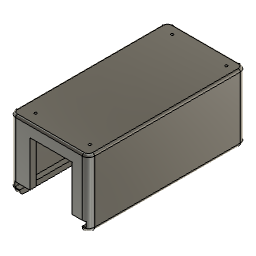
Accelerator UTP v8 (Autodesk Fusion 360 design; units mm, degrees)
Autodesk Fusion 360 part; units mm, degrees
sketch "base" plane through (0, 0, 0) normal (0, 0, 1) x (1, 0, 0) in component "Accelerator"
  line L0 (0, 0) -> (38.5, 0)
  line L1 (38.5, 0) -> (38.5, 74)
  line L2 (38.5, 74) -> (0, 74)
  line L3 (0, 74) -> (0, 0)
  line L4 (0, 59) -> (38.5, 59)
  line L5 (0, 19) -> (38.5, 19)
  line L6 (5, 0) -> (5, 74)
  line L7 (35.5, 0) -> (35.5, 74)
  line L8 (5, 0) -> (7, 5.75) construction
  line L9 (35.5, 0) -> (33.5, 5.75) construction
  point P0 (7, 5.75)
  point P1 (33.5, 5.75)
  point P2 (33.5, 72.25)
  point P3 (7, 72.25)
  dimension "d1" = 26.5
  dimension "d2" = 66.5
  dimension "d4" = 74
  dimension "d9" = 19
  dimension "d33" = 5
  dimension "d34" = 3
  dimension "d101" = 5.75
  dimension "d102" = 40
  dimension "d150" = 38.5
  constraint horizontal L0
  constraint vertical L1
  constraint horizontal L2
  constraint vertical L3
  constraint coincident L0.start L3.end
  constraint horizontal P2 P3
  constraint vertical P0 P3
  constraint horizontal P0 P1
  constraint vertical P1 P2
  constraint coincident L3 L4.start
  constraint coincident L1 L4.end
  constraint perpendicular L1 L4
  constraint coincident L3 L5.start
  constraint coincident L1 L5.end
  constraint perpendicular L1 L5
  constraint coincident L0 L6.start
  constraint coincident L2 L6.end
  constraint coincident L0 L7.start
  constraint coincident L2 L7.end
  constraint perpendicular L2 L7
  constraint vertical L6
  constraint coincident P0 L8.end
  constraint coincident P1 L9.end
  constraint equal L8 L9
  measures "d1" distance of P0 P1
  measures "d2" distance of P0 P3
  measures "d4" distance of L0.end L1.end
  measures "d9" distance of L0.end L5.end
  measures "d33" distance of L0.start L6.start
  measures "d34" distance of L0.end L7.start
  measures "d101" vertical distance of L0.start L8.end
  measures "d102" distance of L4.end L5.end
  measures "d150" distance of L1.end L2.end
extrude "Extrude1" add sketch "base" against normal blind 6 contours L0 L5 L6 L7 | L2 L4 L6 L7 makes body 1 at (25.3333, 6.3333, 0) makes body 2 at (25.3333, 64, 0) in component "Accelerator"
extrude "Extrude2" add sketch "base" against normal blind 3 contours L4 L5 L6 L7 bodies 1 2 in component "Accelerator"
extrude "Extrude3" add sketch "base" against normal blind 33 contours L0 L3 L5 L6 | L3 L4 L5 L6 | L0 L1 L5 L7 | L2 L3 L4 L6 | L1 L4 L5 L7 | L1 L2 L4 L7 bodies 1 in component "Accelerator"
hole "Hole1" at (7, 5.75, 0) at (33.5, 5.75, 0) at (7, 72.25, 0) at (33.5, 72.25, 0) direction (0, 0, -1) diameter 1.2 end up to surface (6 mm away) bodies 1 in component "Accelerator"
sketch "bolts" plane through (5, 0, 0) normal (1, 0, 0) x (0, 1, 0) in component "Accelerator"
  line L0 (19, -6) -> (0, -6)
  line L1 (0, -6) -> (0, -33)
  line L2 (0, -33) -> (74, -33)
  line L3 (74, -33) -> (74, -6)
  line L4 (74, -6) -> (59, -6)
  line L5 (59, -6) -> (59, -3)
  line L6 (59, -3) -> (19, -3)
  line L7 (19, -3) -> (19, -6)
  line L8 (0, -33) -> (17, -11) construction
  line L9 (74, -33) -> (57, -11) construction
  line L10 (74, 0) -> (0, 0)
  point P0 (17, -11)
  point P1 (57, -11)
  dimension "d53" = 11
  dimension "d54" = 40
  constraint coincident L1.end L2.start
  constraint coincident P0 L8.end
  constraint coincident L2.end L3.start
  constraint coincident P1 L9.end
  constraint equal L8 L9
  constraint horizontal P0 P1
  measures "d53" distance of P1 L10
  measures "d54" distance of P0 P1
hole "Hole3" at (5, 17, -11) at (5, 57, -11) direction (-1, 0, 0) diameter 5.3 end up to surface (5 mm away) counterbore diameter 10 counterbore depth 3.5 bodies 1 in component "Accelerator"
fillet "Fillet9" radius 6 2 edges at (20.25, 19, -6) (20.25, 59, -6) on bodies 1 in component "Accelerator"
sketch "flatcable-plate" plane through (0, 74, 0) normal (0, 1, 0) x (-1, 0, 0) in component "Accelerator"
  line L0 (0, 0) -> (-38.5, 0)
  line L1 (-38.5, 0) -> (-38.5, -33)
  line L2 (-38.5, -33) -> (-35.5, -33)
  line L3 (-35.5, -33) -> (-35.5, -6)
  line L4 (-35.5, -6) -> (-5, -6)
  line L5 (-5, -6) -> (-5, -33)
  line L6 (-5, -33) -> (0, -33)
  line L7 (0, -33) -> (0, 0)
  line L8 (-38.5, 0) -> (0, 0)
  line L9 (0, 0) -> (0, -33)
  line L10 (0, -33) -> (-38.5, -33)
  line L11 (-38.5, -33) -> (-38.5, 0)
  constraint horizontal L8
  constraint vertical L9
  constraint horizontal L10
  constraint vertical L11
  constraint coincident L6.end L7.start
  constraint coincident L0.end L1.start
extrude "Extrude12" add sketch "flatcable-plate" along normal blind 3 bodies 1 in component "Accelerator"
sketch "lid-uitsnede" plane through (0, 0, 0) normal (0, -1, 0) x (1, 0, 0) in component "Accelerator"
  line L0 (38.5, 0) -> (0, 0)
  line L1 (0, 0) -> (0, -33)
  line L2 (0, -33) -> (5, -33)
  line L3 (5, -33) -> (5, -6)
  line L4 (5, -6) -> (35.5, -6)
  line L5 (35.5, -6) -> (35.5, -33)
  line L6 (35.5, -33) -> (38.5, -33)
  line L7 (38.5, -33) -> (38.5, 0)
  line L8 (2.5, -28.1) -> (37, -28.1)
  line L9 (37, -28.1) -> (37, -30.5)
  line L10 (37, -30.5) -> (2.5, -30.5)
  line L11 (2.5, -30.5) -> (2.5, -28.1)
  line L12 (2.5, -30.5) -> (0, -33) construction
  line L13 (2.5, -30.5) -> (5, -33) construction
  line L14 (37, -30.5) -> (35.5, -33) construction
  line L15 (37, -30.5) -> (38.5, -33) construction
  dimension "d95" = 2.4
  dimension "d97" = 2.5
  constraint horizontal L8
  constraint vertical L9
  constraint horizontal L10
  constraint vertical L11
  constraint coincident L1.end L2.start
  constraint coincident L2.end L3.start
  constraint coincident L5.end L6.start
  constraint coincident L6.end L7.start
  constraint equal L14 L15
  constraint equal L12 L13
  measures "d95" distance of L8.end L9.end
  measures "d97" vertical distance of L10.end L1.end
sketch "flatcable" plane through (0, 74, 0) normal (0, -1, 0) x (1, 0, 0) in component "Accelerator"
  line L0 (35.5, -33) -> (35.5, -6)
  line L1 (35.5, -6) -> (5, -6)
  line L2 (5, -6) -> (5, -33)
  line L3 (5, -33) -> (35.5, -33)
  line L4 (10.25, -10) -> (30.25, -10)
  line L5 (30.25, -10) -> (30.25, -18.5)
  line L6 (30.25, -18.5) -> (10.25, -18.5)
  line L7 (10.25, -18.5) -> (10.25, -10)
  line L8 (35.5, -33) -> (30.25, -18.5) construction
  line L9 (35.5, -6) -> (30.25, -10) construction
  line L10 (10.25, -10) -> (5, -6) construction
  point P0 (5, -6)
  point P1 (35.5, -6)
  point P2 (35.5, -33)
  dimension "d147" = 20
  dimension "d148" = 8.5
  dimension "d149" = 4
  constraint horizontal L4
  constraint vertical L5
  constraint horizontal L6
  constraint vertical L7
  constraint coincident P2 L0.start
  constraint coincident P1 L0.end
  constraint coincident P0 L1.end
  constraint equal L9 L10
  measures "d147" distance of L4.start L4.end
  measures "d148" distance of L4.start L6.end
  measures "d149" vertical distance of L4.end P1
sketch "space" plane through (0, 0, -6) normal (0, 0, -1) x (1, 0, 0) in component "Accelerator"
  line L0 (5, -13.8038) -> (35.5, -13.8038)
  line L1 (35.5, -13.8038) -> (35.5, 0)
  line L2 (35.5, 0) -> (5, 0)
  line L3 (5, 0) -> (5, -13.8038)
  circle A0 centre (7, -5.75) radius 0.6
  circle A1 centre (33.5, -5.75) radius 0.6
  line L4 (5, 0) -> (10, 0)
  line L5 (10, 0) -> (10, -3)
  line L6 (10, -3) -> (5, -3)
  line L7 (5, -3) -> (5, 0)
  line L8 (35.5, 0) -> (30.5, 0)
  line L9 (30.5, 0) -> (30.5, -3)
  line L10 (30.5, -3) -> (35.5, -3)
  line L11 (35.5, -3) -> (35.5, 0)
  dimension "d112" = 5
  dimension "d113" = 3
  constraint horizontal L4
  constraint vertical L5
  constraint horizontal L6
  constraint vertical L7
  constraint coincident L2.end L3.start
  constraint horizontal L8
  constraint vertical L9
  constraint horizontal L10
  constraint vertical L11
  constraint coincident L1.end L2.start
  constraint equal L6 L10
  constraint equal L5 L9
  measures "d112" distance of L5.end L6.end
  measures "d113" distance of L4.end L5.end
extrude "Extrude17" add sketch "space" along normal blind 23 contours L2 L3 L4 L5 L6 L7 | L1 L2 L8 L9 L10 L11 bodies 1 in component "Accelerator"
extrude "Extrude14" cut sketch "lid-uitsnede" against normal blind 75.5 contours L3 L5 L8 L10 | L5 L8 L9 L10 | L3 L8 L10 L11 bodies 1 in component "Accelerator"
fillet "Fillet14" radius 3 4 edges at (38.5, 0, -16.5) (0, 0, -16.5) (38.5, 77, -16.5) (0, 77, -16.5) on bodies 1 in component "Accelerator"
fillet "Fillet15" radius 1 8 edges at (0.8787, 0.8787, 0) (19.25, 0, 0) (37.6213, 0.8787, 0) (38.5, 38.5, 0) (37.6213, 76.1213, 0) (19.25, 77, 0) (0.8787, 76.1213, 0) (0, 38.5, 0) on bodies 1 in component "Accelerator"
fillet "Fillet16" radius 2 8 edges at (4, 0, -33) (0.8787, 0.8787, -33) (0, 38.5, -33) (0.8787, 76.1213, -33) (19.25, 77, -33) (37.6213, 76.1213, -33) (38.5, 38.5, -33) (37.6213, 0.8787, -33) on bodies 1 in component "Accelerator"
sketch "lid" plane through (0, 0, -5.9316) normal (0, 0, -1) x (1, 0, 0) in component "Lid"
  line L0 (30.5892, -2.7578) -> (30.5892, 0.2422)
  line L1 (30.5892, 0.2422) -> (10.0892, 0.2422)
  line L2 (10.0892, 0.2422) -> (10.0892, -2.7578)
  line L3 (0.0892, 0.2422) -> (34.0892, 0.2422)
  line L4 (34.0892, 0.2422) -> (34.0892, -74.7578)
  line L5 (34.0892, -74.7578) -> (0.0892, -74.7578)
  line L6 (0.0892, -74.7578) -> (0.0892, 0.2422)
  point P0 (0.0892, 0.2422)
  dimension "d171" = 34
  dimension "d172" = 75
  constraint horizontal L3
  constraint vertical L4
  constraint horizontal L5
  constraint vertical L6
  constraint coincident P0 L3.start
  measures "d171" distance of P0 L3.end
  measures "d172" distance of P0 L5.end
extrude "Extrude23" cut sketch "flatcable" against normal up to surface (3 mm away) contours L4 L5 L6 L7 bodies 1 in component "Accelerator"
extrude "Extrude2'" add sketch "lid" along normal blind 1.8 separate body makes body 3 in component "Lid"
fillet "Fillet5" radius 3 2 edges at (34.0892, -0.2422, -6.8316) (0.0892, -0.2422, -6.8316) on bodies 3 in component "Lid"
fillet "Fillet6" radius 0.2 1 faces at (11.4225, 50.7578, -7.7316) on bodies 3 in component "Lid"
fillet "Fillet7" radius 0.2 1 faces at (11.4225, 50.7578, -5.9316) on bodies 3 in component "Lid"
move_body "Move2" bodies 3 to x (1, 0, 0) y (0, 1, 0) z (0, 0, 1) at (0, -85, -54) in component "Lid"
component "Accelerator" placed x (1, 0, 0) y (0, 1, 0) z (0, 0, 1) at (0.0892, -0.2422, 0.0684)
component "Lid" placed x (1, 0, 0) y (0, 1, 0) z (0, 0, 1) at (0, 0, 0)
equation "d4 = base_length"
equation "d100 = -uitsnede"
equation "base_width = 38.5 mm"
equation "base_length = 74 mm"
equation "d150 = base_width"
equation "uitsnede = base_length + 1.5 mm"
equation "lid_width = 34 mm"
equation "d171 = lid_width"
equation "d172 = lid_length"
equation "lid_length = 75 mm"
named bodies: "accelerator-UTP", "accelerator-UTP-LID"
